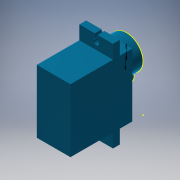
# Autodesk Inventor part: Small continuous Servo Body
Saved by Autodesk Inventor 2016 SP2 (Build 200236200, 236)
## iProperties
Created: 2015-07-13
Part Number: Small continuous Servo Body
Material: ABS Plastic
Document SubType Name: Modeling
Designer: Jared
Density: 1.06 g/cm^3
Appearance: Sky Blue Dark
Mass: 7.49838 g
Surface Area: 26.2443 cm^2
Volume: 7.07394 cm^3
Author: Jared
Autodesk Inventor part; units mm, degrees
ref_plane "YZ Plane" through (0, 0, 0) normal (1, 0, 0) x (0, 1, 0)
ref_plane "XZ Plane" through (0, 0, 0) normal (0, 1, 0) x (-1, 0, 0)
sketch "Sketch1" plane through (0, 0, 0) normal (0, 1, 0) x (-1, 0, 0)
  line L0 (0, 0) -> (12.25, 0)
  line L1 (12.25, 0) -> (12.25, 23)
  line L2 (12.25, 23) -> (0, 23)
  line L3 (0, 23) -> (0, 0)
  dimension "d0" = 12.25
  dimension "d1" = 23
  constraints: 8 end point, 3 perpendicular, 1 horizontal
  measures "d0" distance of L0.start L0.end
  measures "d1" distance of L0.end L1.end
extrude "Extrusion1" add sketch "Sketch1" along normal blind 22.5
sketch "Sketch2" plane through (-12.25, 0, 23) normal (0, 0, 1) x (1, 0, 0)
  line L0 (0, 0) -> (12.25, 0) projected
  line L1 (12.25, 0) -> (12.25, 22.5) projected
  line L2 (0, 22.5) -> (12.25, 22.5) projected
  line L3 (0, 0) -> (0, 22.5) projected
  line L4 (12.25, 22.5) -> (12.25, 18)
  line L5 (12.25, 0) -> (12.25, 22.5) projected
  line L6 (0, 0) -> (0, 22.5) projected
  line L7 (12.25, 18) -> (0, 18)
  line L8 (0, 18) -> (0, 15.5)
  line L9 (0, 15.5) -> (12.25, 15.5)
  dimension "d4" = 4.5
  dimension "d5" = 2.5
  constraints: 8 end point, 4 point on line, 2 perpendicular
  measures "d4" distance of L1.end L4.end
  measures "d5" distance of L7.end L8.end
extrude "Extrusion2" add sketch "Sketch2" along normal blind 5 contours L3 L7 L1 L9
sketch "Sketch3" plane through (-12.25, 18, 23) normal (0, 1, 0) x (1, 0, 0)
  line L0 (0, 0) -> (12.25, 0) projected
  line L1 (0, 0) -> (0, -5) projected
  line L2 (12.25, -5) -> (0, -5) projected
  line L3 (12.25, 0) -> (12.25, -5) projected
  line L4 (0, -5) -> (12.25, -5) projected
  line L5 (6.125, -1.5) -> (6.125, 0)
  line L6 (6.125, -5) -> (5.625, -5)
  line L7 (5.625, -5) -> (5.625, -3.366)
  arc A0 (6.125, -1.5) -> (5.625, -3.366) centre (6.125, -2.5) ccw
  line L8 (6.625, -5) -> (6.625, -3.366)
  arc A1 (6.625, -3.366) -> (6.125, -1.5) centre (6.125, -2.5) ccw
  line L9 (6.625, -5) -> (6.125, -5)
  point P0 (12.25, 23)
  dimension "d8" = 0.5
  dimension "d9" = 2
  dimension "d10" = 0.5
  dimension "d11" = 3.5
  constraints: 10 end point, 4 point on circle, 2 centre point, 2 midpoint, 2 point on line, 2 symmetric about line, 1 perpendicular, 1 other
  measures "d8" distance of L6.start L6.end
  measures "d9" diameter of A0
  measures "d10" distance of L6.start L8.start
  measures "d11" distance of L6.start L5.start
extrude "Extrusion3" cut sketch "Sketch3" against normal up to next contours A1 L8 L2 L7 A0
ref_plane "Work Plane1" through (-12.25, 0, 11.5) normal (0, 0, 1) x (1, 0, 0)
mirror "Mirror1" about plane through (-12.25, 0, 11.5) normal (0, 0, 1) of "Extrusion2", "Extrusion3"
sketch "Sketch4" plane through (0, 22.5, 0) normal (0, 1, 0) x (1, 0, 0)
  line L0 (0, 0) -> (-12.25, 0) projected
  line L1 (-12.25, 0) -> (-12.25, -23) projected
  line L2 (-12.25, -23) -> (0, -23) projected
  line L3 (0, -23) -> (0, 0) projected
  line L4 (-12.25, -23) -> (0, -23) projected
  line L5 (-6.125, -23) -> (-6.125, -17)
  arc A0 (-8.6615, -11.5625) -> (-3.5885, -11.5625) centre (-6.125, -17) ccw
  line L6 (-6.125, -17) -> (-6.125, -10.5)
  arc A1 (-3.5885, -11.5625) -> (-8.6615, -11.5625) centre (-6.125, -10.5) ccw
  dimension "d14" = 6
  dimension "d15" = 6.5
  dimension "d16" = 5.5
  constraints: 5 point on circle, 4 end point, 2 centre point, 2 coincident, 2 vertical, 1 midpoint
  measures "d14" distance of L5.start L5.end
  measures "d15" distance of L6.start L6.end
  measures "d16" diameter of A1
extrude "Extrusion4" add sketch "Sketch4" along normal blind 4 contours A0 A1
sketch "Sketch5" plane through (0, 26.5, 0) normal (0, 1, 0) x (1, 0, 0)
  arc A0 (-8.6615, -11.5625) -> (-3.5885, -11.5625) centre (-6.125, -17) ccw projected
  arc A1 (-3.5885, -11.5625) -> (-8.6615, -11.5625) centre (-6.125, -10.5) ccw projected
  arc A2 (-3.5885, -11.5625) -> (-8.6615, -11.5625) centre (-6.125, -17) ccw
  circle A3 centre (-6.125, -17) radius 2.5
  arc A4 (-3.5885, -11.5625) -> (-8.6615, -11.5625) centre (-6.125, -10.5) ccw projected
  arc A5 (-8.6615, -11.5625) -> (-3.5885, -11.5625) centre (-6.125, -17) ccw projected
  point P0 (0, 0)
  dimension "d19" = 6
  dimension "d20" = 5
  constraints: 2 centre point, 2 point on circle, 1 coincident
  measures "d19" radius of A2
  measures "d20" diameter of A3
body "Solid1"
